Autodesk Fusion 360 part; units mm, degrees
(part 18 of 20)
  spline S542 degree 3 poles (32.1624, -86.398) (32.3125, -86.213) (32.6036, -85.8545) (33.0601, -85.7933) (33.281, -85.7636) knots 0 0 0 0 0.068625 0.133023 0.133023 0.133023 0.133023
  spline S543 degree 3 poles (33.281, -85.7636) (33.4461, -85.772) (33.754, -85.7877) (33.9971, -85.9751) (34.1098, -86.0621) knots 0 0 0 0 0.048244 0.08997 0.08997 0.08997 0.08997
  spline S544 degree 3 poles (34.1098, -86.0621) (34.1941, -86.1844) (34.3835, -86.4593) (34.394, -86.7949) (34.3997, -86.9812) knots 0 0 0 0 0.043695 0.098195 0.098195 0.098195 0.098195
  line L449 (34.3997, -86.9812) -> (34.3997, -89.4676)
  line L450 (34.3997, -89.4676) -> (33.7892, -89.4676)
  line L451 (33.7892, -89.4676) -> (33.7892, -87.1859)
  spline S545 degree 3 poles (33.7892, -87.1859) (33.7892, -87.0797) (33.7892, -86.9003) (33.7468, -86.7264) (33.7295, -86.6555) knots 0 0 0 0 0.031711 0.053535 0.053535 0.053535 0.053535
  spline S546 degree 3 poles (33.7295, -86.6555) (33.7051, -86.6038) (33.6553, -86.4984) (33.561, -86.4297) (33.513, -86.3946) knots 0 0 0 0 0.016863 0.034394 0.034394 0.034394 0.034394
  spline S547 degree 3 poles (33.513, -86.3946) (33.4572, -86.3658) (33.3418, -86.306) (33.2118, -86.2992) (33.1446, -86.2957) knots 0 0 0 0 0.018597 0.038532 0.038532 0.038532 0.038532
  spline S548 degree 3 poles (33.1446, -86.2957) (33.0235, -86.3055) (32.7855, -86.3247) (32.6009, -86.4757) (32.5102, -86.5498) knots 0 0 0 0 0.035532 0.069798 0.069798 0.069798 0.069798
  spline S549 degree 3 poles (32.5102, -86.5498) (32.4369, -86.6565) (32.2698, -86.8996) (32.2621, -87.1966) (32.2578, -87.3632) knots 0 0 0 0 0.038079 0.086792 0.086792 0.086792 0.086792
  line L452 (32.2578, -87.3632) -> (32.2579, -89.4676)
  line L453 (32.2579, -89.4676) -> (31.6439, -89.4676)
  line L454 (31.6439, -89.4676) -> (31.6439, -87.1142)
  spline S550 degree 3 poles (31.6439, -87.1142) (31.6415, -86.9922) (31.6372, -86.7754) (31.5375, -86.584) (31.4939, -86.5003) knots 0 0 0 0 0.036008 0.063954 0.063954 0.063954 0.063954
  spline S551 degree 3 poles (31.4939, -86.5003) (31.4316, -86.4408) (31.2954, -86.3104) (31.1058, -86.3009) (31.0027, -86.2957) knots 0 0 0 0 0.025037 0.054812 0.054812 0.054812 0.054812
  spline S552 degree 3 poles (31.0027, -86.2957) (30.918, -86.3014) (30.7485, -86.3127) (30.5985, -86.3923) (30.5235, -86.4321) knots 0 0 0 0 0.025172 0.050327 0.050327 0.050327 0.050327
  spline S553 degree 3 poles (30.5235, -86.4321) (30.4549, -86.4838) (30.3146, -86.5894) (30.2418, -86.7494) (30.2046, -86.8312) knots 0 0 0 0 0.025339 0.051812 0.051812 0.051812 0.051812
  spline S554 degree 3 poles (30.2046, -86.8312) (30.1759, -86.9375) (30.1091, -87.185) (30.107, -87.4418) (30.1057, -87.5883) knots 0 0 0 0 0.032907 0.076633 0.076633 0.076633 0.076633
  line L455 (30.1057, -87.5883) -> (30.1057, -89.4676)
  line L456 (30.1057, -89.4676) -> (29.4918, -89.4676)
  line L457 (18.1003, -85.1224) -> (18.1003, -84.5324)
  line L458 (18.1003, -84.5324) -> (21.337, -84.5324)
  line L459 (21.337, -84.5324) -> (21.337, -85.0099)
  spline S555 degree 3 poles (21.337, -85.0099) (21.1728, -85.2031) (20.8154, -85.6236) (20.5396, -86.1019) (20.3905, -86.3605) knots 0 0 0 0 0.075903 0.165223 0.165223 0.165223 0.165223
  spline S556 degree 3 poles (20.3905, -86.3605) (20.2435, -86.6418) (19.9525, -87.1986) (19.7607, -87.797) (19.6658, -88.0931) knots 0 0 0 0 0.095012 0.188116 0.188116 0.188116 0.188116
  spline S557 degree 3 poles (19.6658, -88.0931) (19.6097, -88.3112) (19.4935, -88.7629) (19.4519, -89.2274) (19.4304, -89.4676) knots 0 0 0 0 0.06745 0.139654 0.139654 0.139654 0.139654
  line L460 (19.4304, -89.4676) -> (18.7995, -89.4676)
  spline S558 degree 3 poles (18.7995, -89.4676) (18.8147, -89.2495) (18.8485, -88.7675) (18.9667, -88.2987) (19.0314, -88.0419) knots 0 0 0 0 0.065448 0.144689 0.144689 0.144689 0.144689
  spline S559 degree 3 poles (19.0314, -88.0419) (19.1136, -87.7653) (19.2788, -87.2097) (19.5375, -86.6909) (19.6675, -86.4304) knots 0 0 0 0 0.086392 0.173544 0.173544 0.173544 0.173544
  spline S560 degree 3 poles (19.6675, -86.4304) (19.8031, -86.1874) (20.0603, -85.7265) (20.3922, -85.3163) (20.5491, -85.1224) knots 0 0 0 0 0.083307 0.157996 0.157996 0.157996 0.157996
  line L461 (20.5491, -85.1224) -> (18.1003, -85.1224)
  line L462 (29.4918, -139.5) -> (29.4918, -135.8779)
  line L463 (29.4918, -135.8779) -> (30.0409, -135.8779)
  line L464 (30.0409, -135.8779) -> (30.0409, -136.3861)
  spline S561 degree 3 poles (30.0409, -136.3861) (30.1028, -136.3015) (30.2277, -136.131) (30.4051, -136.016) (30.4945, -135.9581) knots 0 0 0 0 0.031158 0.062835 0.062835 0.062835 0.062835
  spline S562 degree 3 poles (30.4945, -135.9581) (30.5937, -135.9108) (30.7976, -135.8137) (31.0232, -135.802) (31.1391, -135.7961) knots 0 0 0 0 0.032617 0.067048 0.067048 0.067048 0.067048
  spline S563 degree 3 poles (31.1391, -135.7961) (31.2636, -135.8008) (31.496, -135.8096) (31.703, -135.9145) (31.7991, -135.9632) knots 0 0 0 0 0.036859 0.068796 0.068796 0.068796 0.068796
  spline S564 degree 3 poles (31.7991, -135.9632) (31.8788, -136.0249) (32.0397, -136.1496) (32.1212, -136.3362) (32.1623, -136.4304) knots 0 0 0 0 0.029725 0.060035 0.060035 0.060035 0.060035
  spline S565 degree 3 poles (32.1623, -136.4304) (32.3125, -136.2455) (32.6036, -135.8869) (33.0601, -135.8257) (33.281, -135.7961) knots 0 0 0 0 0.068625 0.133023 0.133023 0.133023 0.133023
  spline S566 degree 3 poles (33.281, -135.7961) (33.4461, -135.8045) (33.754, -135.8201) (33.9971, -136.0076) (34.1098, -136.0945) knots 0 0 0 0 0.048244 0.08997 0.08997 0.08997 0.08997
  spline S567 degree 3 poles (34.1098, -136.0945) (34.1941, -136.2168) (34.3835, -136.4917) (34.3939, -136.8274) (34.3997, -137.0137) knots 0 0 0 0 0.043695 0.098195 0.098195 0.098195 0.098195
  line L465 (34.3997, -137.0137) -> (34.3997, -139.5)
  line L466 (34.3997, -139.5) -> (33.7892, -139.5)
  line L467 (33.7892, -139.5) -> (33.7892, -137.2183)
  spline S568 degree 3 poles (33.7892, -137.2183) (33.7892, -137.1121) (33.7891, -136.9328) (33.7468, -136.7588) (33.7295, -136.6879) knots 0 0 0 0 0.031711 0.053535 0.053535 0.053535 0.053535
  spline S569 degree 3 poles (33.7295, -136.6879) (33.7051, -136.6363) (33.6552, -136.5309) (33.561, -136.4621) (33.5129, -136.427) knots 0 0 0 0 0.016863 0.034394 0.034394 0.034394 0.034394
  spline S570 degree 3 poles (33.5129, -136.427) (33.4572, -136.3982) (33.3418, -136.3384) (33.2118, -136.3316) (33.1446, -136.3281) knots 0 0 0 0 0.018597 0.038532 0.038532 0.038532 0.038532
  spline S571 degree 3 poles (33.1446, -136.3281) (33.0235, -136.3379) (32.7855, -136.3572) (32.6009, -136.5081) (32.5102, -136.5822) knots 0 0 0 0 0.035532 0.069798 0.069798 0.069798 0.069798
  spline S572 degree 3 poles (32.5102, -136.5822) (32.4369, -136.6889) (32.2697, -136.9321) (32.2621, -137.229) (32.2578, -137.3956) knots 0 0 0 0 0.038079 0.086792 0.086792 0.086792 0.086792
  line L468 (32.2578, -137.3956) -> (32.2578, -139.5)
  line L469 (32.2578, -139.5) -> (31.6439, -139.5)
  line L470 (31.6439, -139.5) -> (31.6439, -137.1467)
  spline S573 degree 3 poles (31.6439, -137.1467) (31.6415, -137.0246) (31.6372, -136.8078) (31.5374, -136.6164) (31.4938, -136.5328) knots 0 0 0 0 0.036008 0.063954 0.063954 0.063954 0.063954
  spline S574 degree 3 poles (31.4938, -136.5328) (31.4316, -136.4732) (31.2954, -136.3428) (31.1057, -136.3333) (31.0027, -136.3281) knots 0 0 0 0 0.025037 0.054812 0.054812 0.054812 0.054812
  spline S575 degree 3 poles (31.0027, -136.3281) (30.918, -136.3338) (30.7485, -136.3451) (30.5985, -136.4247) (30.5235, -136.4645) knots 0 0 0 0 0.025172 0.050327 0.050327 0.050327 0.050327
  spline S576 degree 3 poles (30.5235, -136.4645) (30.4549, -136.5162) (30.3146, -136.6218) (30.2418, -136.7818) (30.2046, -136.8636) knots 0 0 0 0 0.025339 0.051812 0.051812 0.051812 0.051812
  spline S577 degree 3 poles (30.2046, -136.8636) (30.1759, -136.9699) (30.1091, -137.2174) (30.1069, -137.4742) (30.1057, -137.6207) knots 0 0 0 0 0.032907 0.076633 0.076633 0.076633 0.076633
  line L471 (30.1057, -137.6207) -> (30.1057, -139.5)
  line L472 (30.1057, -139.5) -> (29.4918, -139.5)
  line L473 (18.1003, -135.1548) -> (18.1003, -134.5648)
  line L474 (18.1003, -134.5648) -> (21.337, -134.5648)
  line L475 (21.337, -134.5648) -> (21.337, -135.0423)
  spline S578 degree 3 poles (21.337, -135.0423) (21.1728, -135.2355) (20.8153, -135.656) (20.5396, -136.1343) (20.3905, -136.3929) knots 0 0 0 0 0.075903 0.165223 0.165223 0.165223 0.165223
  spline S579 degree 3 poles (20.3905, -136.3929) (20.2435, -136.6742) (19.9525, -137.2311) (19.7607, -137.8294) (19.6657, -138.1255) knots 0 0 0 0 0.095012 0.188116 0.188116 0.188116 0.188116
  spline S580 degree 3 poles (19.6657, -138.1255) (19.6096, -138.3436) (19.4935, -138.7953) (19.4519, -139.2598) (19.4304, -139.5) knots 0 0 0 0 0.06745 0.139654 0.139654 0.139654 0.139654
  line L476 (19.4304, -139.5) -> (18.7994, -139.5)
  spline S581 degree 3 poles (18.7994, -139.5) (18.8147, -139.282) (18.8485, -138.7999) (18.9666, -138.3311) (19.0314, -138.0744) knots 0 0 0 0 0.065448 0.144689 0.144689 0.144689 0.144689
  spline S582 degree 3 poles (19.0314, -138.0744) (19.1136, -137.7977) (19.2788, -137.2421) (19.5375, -136.7233) (19.6674, -136.4628) knots 0 0 0 0 0.086392 0.173544 0.173544 0.173544 0.173544
  spline S583 degree 3 poles (19.6674, -136.4628) (19.8031, -136.2198) (20.0602, -135.7589) (20.3922, -135.3487) (20.5491, -135.1548) knots 0 0 0 0 0.083307 0.157996 0.157996 0.157996 0.157996
  line L477 (20.5491, -135.1548) -> (18.1003, -135.1548)
  line L478 (29.5259, -189.5) -> (29.5259, -185.8779)
  line L479 (29.5259, -185.8779) -> (30.075, -185.8779)
  line L480 (30.075, -185.8779) -> (30.075, -186.3861)
  spline S584 degree 3 poles (30.075, -186.3861) (30.137, -186.3015) (30.2618, -186.131) (30.4392, -186.016) (30.5287, -185.958) knots 0 0 0 0 0.031158 0.062835 0.062835 0.062835 0.062835
  spline S585 degree 3 poles (30.5287, -185.958) (30.6278, -185.9108) (30.8317, -185.8137) (31.0574, -185.802) (31.1733, -185.796) knots 0 0 0 0 0.032617 0.067048 0.067048 0.067048 0.067048
  spline S586 degree 3 poles (31.1733, -185.796) (31.2978, -185.8008) (31.5301, -185.8096) (31.7371, -185.9145) (31.8332, -185.9632) knots 0 0 0 0 0.036859 0.068796 0.068796 0.068796 0.068796
  spline S587 degree 3 poles (31.8332, -185.9632) (31.9129, -186.0249) (32.0738, -186.1496) (32.1553, -186.3362) (32.1965, -186.4304) knots 0 0 0 0 0.029725 0.060035 0.060035 0.060035 0.060035
  spline S588 degree 3 poles (32.1965, -186.4304) (32.3466, -186.2454) (32.6378, -185.8869) (33.0942, -185.8257) (33.3151, -185.796) knots 0 0 0 0 0.068625 0.133023 0.133023 0.133023 0.133023
  spline S589 degree 3 poles (33.3151, -185.796) (33.4802, -185.8045) (33.7881, -185.8201) (34.0312, -186.0076) (34.1439, -186.0945) knots 0 0 0 0 0.048244 0.08997 0.08997 0.08997 0.08997
  spline S590 degree 3 poles (34.1439, -186.0945) (34.2282, -186.2168) (34.4177, -186.4917) (34.4281, -186.8273) (34.4338, -187.0136) knots 0 0 0 0 0.043695 0.098195 0.098195 0.098195 0.098195
  line L481 (34.4338, -187.0136) -> (34.4338, -189.5)
  line L482 (34.4338, -189.5) -> (33.8233, -189.5)
  line L483 (33.8233, -189.5) -> (33.8233, -187.2183)
  spline S591 degree 3 poles (33.8233, -187.2183) (33.8233, -187.1121) (33.8233, -186.9327) (33.7809, -186.7588) (33.7636, -186.6879) knots 0 0 0 0 0.031711 0.053535 0.053535 0.053535 0.053535
  spline S592 degree 3 poles (33.7636, -186.6879) (33.7392, -186.6362) (33.6894, -186.5308) (33.5951, -186.4621) (33.5471, -186.427) knots 0 0 0 0 0.016863 0.034394 0.034394 0.034394 0.034394
  spline S593 degree 3 poles (33.5471, -186.427) (33.4914, -186.3982) (33.3759, -186.3384) (33.246, -186.3316) (33.1787, -186.3281) knots 0 0 0 0 0.018597 0.038532 0.038532 0.038532 0.038532
  spline S594 degree 3 poles (33.1787, -186.3281) (33.0576, -186.3379) (32.8196, -186.3571) (32.635, -186.5081) (32.5443, -186.5822) knots 0 0 0 0 0.035532 0.069798 0.069798 0.069798 0.069798
  spline S595 degree 3 poles (32.5443, -186.5822) (32.471, -186.6889) (32.3039, -186.932) (32.2962, -187.229) (32.292, -187.3956) knots 0 0 0 0 0.038079 0.086792 0.086792 0.086792 0.086792
  line L484 (32.292, -187.3956) -> (32.292, -189.5)
  line L485 (32.292, -189.5) -> (31.678, -189.5)
  line L486 (31.678, -189.5) -> (31.678, -187.1467)
  spline S596 degree 3 poles (31.678, -187.1467) (31.6756, -187.0246) (31.6713, -186.8078) (31.5716, -186.6164) (31.528, -186.5327) knots 0 0 0 0 0.036008 0.063954 0.063954 0.063954 0.063954
  spline S597 degree 3 poles (31.528, -186.5327) (31.4658, -186.4732) (31.3295, -186.3428) (31.1399, -186.3333) (31.0368, -186.3281) knots 0 0 0 0 0.025037 0.054812 0.054812 0.054812 0.054812
  spline S598 degree 3 poles (31.0368, -186.3281) (30.9521, -186.3338) (30.7826, -186.3451) (30.6326, -186.4247) (30.5576, -186.4645) knots 0 0 0 0 0.025172 0.050327 0.050327 0.050327 0.050327
  spline S599 degree 3 poles (30.5576, -186.4645) (30.489, -186.5162) (30.3487, -186.6218) (30.2759, -186.7818) (30.2388, -186.8636) knots 0 0 0 0 0.025339 0.051812 0.051812 0.051812 0.051812
  spline S600 degree 3 poles (30.2388, -186.8636) (30.21, -186.9699) (30.1432, -187.2174) (30.1411, -187.4742) (30.1398, -187.6207) knots 0 0 0 0 0.032907 0.076633 0.076633 0.076633 0.076633
  line L487 (30.1398, -187.6207) -> (30.1398, -189.5)
  line L488 (30.1398, -189.5) -> (29.5259, -189.5)
  line L489 (21.279, -185.7244) -> (20.6685, -185.7722)
  spline S601 degree 3 poles (20.6685, -185.7722) (20.6425, -185.6649) (20.5967, -185.4753) (20.485, -185.3161) (20.4366, -185.2469) knots 0 0 0 0 0.032737 0.057863 0.057863 0.057863 0.057863
  spline S602 degree 3 poles (20.4366, -185.2469) (20.3486, -185.1703) (20.1722, -185.0168) (19.9394, -184.9952) (19.8227, -184.9843) knots 0 0 0 0 0.034068 0.068298 0.068298 0.068298 0.068298
  spline S603 degree 3 poles (19.8227, -184.9843) (19.7285, -184.9907) (19.5433, -185.0032) (19.3853, -185.1003) (19.3076, -185.148) knots 0 0 0 0 0.027843 0.054766 0.054766 0.054766 0.054766
  spline S604 degree 3 poles (19.3076, -185.148) (19.2148, -185.2299) (19.0188, -185.4028) (18.9086, -185.6403) (18.8506, -185.7654) knots 0 0 0 0 0.036718 0.077555 0.077555 0.077555 0.077555
  spline S605 degree 3 poles (18.8506, -185.7654) (18.8017, -185.9283) (18.6886, -186.3047) (18.681, -186.6983) (18.6767, -186.9216) knots 0 0 0 0 0.050812 0.1174 0.1174 0.1174 0.1174
  spline S606 degree 3 poles (18.6767, -186.9216) (18.753, -186.8171) (18.9011, -186.6144) (19.1152, -186.4836) (19.219, -186.4202) knots 0 0 0 0 0.038374 0.074495 0.074495 0.074495 0.074495
  spline S607 degree 3 poles (19.219, -186.4202) (19.3267, -186.3724) (19.5409, -186.2776) (19.7747, -186.2635) (19.8909, -186.2565) knots 0 0 0 0 0.035048 0.069654 0.069654 0.069654 0.069654
  spline S608 degree 3 poles (19.8909, -186.2565) (20.0883, -186.2757) (20.485, -186.3143) (20.7853, -186.5766) (20.9362, -186.7084) knots 0 0 0 0 0.057942 0.116462 0.116462 0.116462 0.116462
  spline S609 degree 3 poles (20.9362, -186.7084) (21.062, -186.8743) (21.3235, -187.2192) (21.3526, -187.6519) (21.3677, -187.8765) knots 0 0 0 0 0.061076 0.12698 0.12698 0.12698 0.12698
  spline S610 degree 3 poles (21.3677, -187.8765) (21.3596, -188.0299) (21.3435, -188.3336) (21.2239, -188.6131) (21.1647, -188.7514) knots 0 0 0 0 0.045687 0.090433 0.090433 0.090433 0.090433
  spline S611 degree 3 poles (21.1647, -188.7514) (21.0922, -188.8773) (20.9503, -189.1236) (20.7197, -189.2894) (20.6071, -189.3704) knots 0 0 0 0 0.043053 0.084173 0.084173 0.084173 0.084173
  spline S612 degree 3 poles (20.6071, -189.3704) (20.4833, -189.4331) (20.2303, -189.5612) (19.9469, -189.5771) (19.8022, -189.5853) knots 0 0 0 0 0.041145 0.084115 0.084115 0.084115 0.084115
  spline S613 degree 3 poles (19.8022, -189.5853) (19.5589, -189.5626) (19.0767, -189.5177) (18.7248, -189.1854) (18.5505, -189.0208) knots 0 0 0 0 0.071077 0.140887 0.140887 0.140887 0.140887
  spline S614 degree 3 poles (18.5505, -189.0208) (18.41, -188.7773) (18.0802, -188.2056) (18.0713, -187.5415) (18.0662, -187.1603) knots 0 0 0 0 0.083095 0.195067 0.195067 0.195067 0.195067
  spline S615 degree 3 poles (18.0662, -187.1603) (18.0727, -186.7324) (18.084, -185.9831) (18.4463, -185.3319) (18.6016, -185.0525) knots 0 0 0 0 0.125884 0.220443 0.220443 0.220443 0.220443
  spline S616 degree 3 poles (18.6016, -185.0525) (18.7734, -184.8854) (19.1238, -184.5445) (19.6115, -184.5015) (19.8602, -184.4795) knots 0 0 0 0 0.069661 0.142118 0.142118 0.142118 0.142118
  spline S617 degree 3 poles (19.8602, -184.4795) (20.0449, -184.4907) (20.3984, -184.512) (20.6885, -184.7139) (20.8271, -184.8104) knots 0 0 0 0 0.054308 0.103968 0.103968 0.103968 0.103968
  spline S618 degree 3 poles (20.8271, -184.8104) (20.9406, -184.9351) (21.178, -185.196) (21.2444, -185.5432) (21.279, -185.7244) knots 0 0 0 0 0.049602 0.103747 0.103747 0.103747 0.103747
  line L490 (29.5256, -239.5001) -> (29.5256, -235.878)
  line L491 (29.5256, -235.878) -> (30.0747, -235.878)
  line L492 (30.0747, -235.878) -> (30.0747, -236.3862)
  spline S619 degree 3 poles (30.0747, -236.3862) (30.1366, -236.3016) (30.2615, -236.1311) (30.4389, -236.0161) (30.5283, -235.9582) knots 0 0 0 0 0.031158 0.062835 0.062835 0.062835 0.062835
  spline S620 degree 3 poles (30.5283, -235.9582) (30.6275, -235.9109) (30.8314, -235.8138) (31.0571, -235.8022) (31.173, -235.7962) knots 0 0 0 0 0.032617 0.067048 0.067048 0.067048 0.067048
  spline S621 degree 3 poles (31.173, -235.7962) (31.2975, -235.8009) (31.5298, -235.8098) (31.7368, -235.9146) (31.8329, -235.9633) knots 0 0 0 0 0.036859 0.068796 0.068796 0.068796 0.068796
  spline S622 degree 3 poles (31.8329, -235.9633) (31.9126, -236.025) (32.0735, -236.1497) (32.155, -236.3363) (32.1961, -236.4305) knots 0 0 0 0 0.029725 0.060035 0.060035 0.060035 0.060035
  spline S623 degree 3 poles (32.1961, -236.4305) (32.3463, -236.2456) (32.6374, -235.887) (33.0939, -235.8258) (33.3148, -235.7962) knots 0 0 0 0 0.068625 0.133023 0.133023 0.133023 0.133023
  spline S624 degree 3 poles (33.3148, -235.7962) (33.4799, -235.8046) (33.7878, -235.8203) (34.0309, -236.0077) (34.1436, -236.0946) knots 0 0 0 0 0.048244 0.08997 0.08997 0.08997 0.08997
  spline S625 degree 3 poles (34.1436, -236.0946) (34.2279, -236.2169) (34.4173, -236.4919) (34.4277, -236.8275) (34.4335, -237.0138) knots 0 0 0 0 0.043695 0.098195 0.098195 0.098195 0.098195
  line L493 (34.4335, -237.0138) -> (34.4335, -239.5001)
  line L494 (34.4335, -239.5001) -> (33.823, -239.5001)
  line L495 (33.823, -239.5001) -> (33.823, -237.2184)
  spline S626 degree 3 poles (33.823, -237.2184) (33.823, -237.1122) (33.8229, -236.9329) (33.7806, -236.759) (33.7633, -236.6881) knots 0 0 0 0 0.031711 0.053535 0.053535 0.053535 0.053535
  spline S627 degree 3 poles (33.7633, -236.6881) (33.7389, -236.6364) (33.6891, -236.531) (33.5948, -236.4622) (33.5468, -236.4271) knots 0 0 0 0 0.016863 0.034394 0.034394 0.034394 0.034394
  spline S628 degree 3 poles (33.5468, -236.4271) (33.491, -236.3983) (33.3756, -236.3386) (33.2456, -236.3318) (33.1784, -236.3282) knots 0 0 0 0 0.018597 0.038532 0.038532 0.038532 0.038532
  spline S629 degree 3 poles (33.1784, -236.3282) (33.0573, -236.338) (32.8193, -236.3573) (32.6347, -236.5082) (32.544, -236.5823) knots 0 0 0 0 0.035532 0.069798 0.069798 0.069798 0.069798
  spline S630 degree 3 poles (32.544, -236.5823) (32.4707, -236.689) (32.3035, -236.9322) (32.2959, -237.2291) (32.2916, -237.3958) knots 0 0 0 0 0.038079 0.086792 0.086792 0.086792 0.086792
  line L496 (32.2916, -237.3958) -> (32.2916, -239.5001)
  line L497 (32.2916, -239.5001) -> (31.6777, -239.5001)
  line L498 (31.6777, -239.5001) -> (31.6777, -237.1468)
  spline S631 degree 3 poles (31.6777, -237.1468) (31.6753, -237.0247) (31.671, -236.808) (31.5713, -236.6165) (31.5277, -236.5329) knots 0 0 0 0 0.036008 0.063954 0.063954 0.063954 0.063954
  spline S632 degree 3 poles (31.5277, -236.5329) (31.4654, -236.4733) (31.3292, -236.3429) (31.1396, -236.3334) (31.0365, -236.3282) knots 0 0 0 0 0.025037 0.054812 0.054812 0.054812 0.054812
  spline S633 degree 3 poles (31.0365, -236.3282) (30.9518, -236.3339) (30.7823, -236.3452) (30.6323, -236.4249) (30.5573, -236.4646) knots 0 0 0 0 0.025172 0.050327 0.050327 0.050327 0.050327
  spline S634 degree 3 poles (30.5573, -236.4646) (30.4887, -236.5163) (30.3484, -236.6219) (30.2756, -236.7819) (30.2384, -236.8637) knots 0 0 0 0 0.025339 0.051812 0.051812 0.051812 0.051812
  spline S635 degree 3 poles (30.2384, -236.8637) (30.2097, -236.97) (30.1429, -237.2175) (30.1407, -237.4743) (30.1395, -237.6208) knots 0 0 0 0 0.032907 0.076633 0.076633 0.076633 0.076633
  line L499 (30.1395, -237.6208) -> (30.1395, -239.5001)
  line L500 (30.1395, -239.5001) -> (29.5256, -239.5001)
  line L501 (21.2787, -235.7245) -> (20.6682, -235.7722)
  spline S636 degree 3 poles (20.6682, -235.7722) (20.6422, -235.6649) (20.5964, -235.4754) (20.4847, -235.3161) (20.4363, -235.247) knots 0 0 0 0 0.032737 0.057863 0.057863 0.057863 0.057863
  spline S637 degree 3 poles (20.4363, -235.247) (20.3483, -235.1704) (20.1719, -235.0168) (19.9391, -234.9952) (19.8223, -234.9843) knots 0 0 0 0 0.034068 0.068298 0.068298 0.068298 0.068298
  spline S638 degree 3 poles (19.8223, -234.9843) (19.7282, -234.9907) (19.543, -235.0032) (19.385, -235.1003) (19.3073, -235.148) knots 0 0 0 0 0.027843 0.054766 0.054766 0.054766 0.054766
  spline S639 degree 3 poles (19.3073, -235.148) (19.2145, -235.2299) (19.0185, -235.4028) (18.9083, -235.6403) (18.8503, -235.7654) knots 0 0 0 0 0.036718 0.077555 0.077555 0.077555 0.077555
  spline S640 degree 3 poles (18.8503, -235.7654) (18.8014, -235.9283) (18.6883, -236.3047) (18.6807, -236.6983) (18.6764, -236.9216) knots 0 0 0 0 0.050812 0.1174 0.1174 0.1174 0.1174
  spline S641 degree 3 poles (18.6764, -236.9216) (18.7527, -236.8172) (18.9008, -236.6145) (19.1149, -236.4836) (19.2187, -236.4202) knots 0 0 0 0 0.038374 0.074495 0.074495 0.074495 0.074495
  spline S642 degree 3 poles (19.2187, -236.4202) (19.3264, -236.3725) (19.5406, -236.2776) (19.7744, -236.2635) (19.8906, -236.2565) knots 0 0 0 0 0.035048 0.069654 0.069654 0.069654 0.069654
  spline S643 degree 3 poles (19.8906, -236.2565) (20.0879, -236.2757) (20.4847, -236.3143) (20.785, -236.5766) (20.9359, -236.7084) knots 0 0 0 0 0.057942 0.116462 0.116462 0.116462 0.116462
  spline S644 degree 3 poles (20.9359, -236.7084) (21.0617, -236.8743) (21.3232, -237.2192) (21.3523, -237.652) (21.3673, -237.8766) knots 0 0 0 0 0.061076 0.12698 0.12698 0.12698 0.12698
  spline S645 degree 3 poles (21.3673, -237.8766) (21.3592, -238.03) (21.3432, -238.3336) (21.2236, -238.6131) (21.1644, -238.7514) knots 0 0 0 0 0.045687 0.090433 0.090433 0.090433 0.090433
  spline S646 degree 3 poles (21.1644, -238.7514) (21.0919, -238.8774) (20.95, -239.1236) (20.7194, -239.2894) (20.6068, -239.3704) knots 0 0 0 0 0.043053 0.084173 0.084173 0.084173 0.084173
  spline S647 degree 3 poles (20.6068, -239.3704) (20.483, -239.4331) (20.2299, -239.5612) (19.9466, -239.5771) (19.8018, -239.5853) knots 0 0 0 0 0.041145 0.084115 0.084115 0.084115 0.084115
  spline S648 degree 3 poles (19.8018, -239.5853) (19.5586, -239.5626) (19.0764, -239.5177) (18.7245, -239.1855) (18.5501, -239.0208) knots 0 0 0 0 0.071077 0.140887 0.140887 0.140887 0.140887
  spline S649 degree 3 poles (18.5501, -239.0208) (18.4097, -238.7773) (18.0799, -238.2056) (18.071, -237.5415) (18.0659, -237.1603) knots 0 0 0 0 0.083095 0.195067 0.195067 0.195067 0.195067
  spline S650 degree 3 poles (18.0659, -237.1603) (18.0723, -236.7324) (18.0837, -235.9831) (18.4459, -235.3319) (18.6013, -235.0525) knots 0 0 0 0 0.125884 0.220443 0.220443 0.220443 0.220443
  spline S651 degree 3 poles (18.6013, -235.0525) (18.7731, -234.8854) (19.1235, -234.5445) (19.6112, -234.5015) (19.8599, -234.4796) knots 0 0 0 0 0.069661 0.142118 0.142118 0.142118 0.142118
  spline S652 degree 3 poles (19.8599, -234.4796) (20.0446, -234.4907) (20.3981, -234.5121) (20.6882, -234.714) (20.8268, -234.8104) knots 0 0 0 0 0.054308 0.103968 0.103968 0.103968 0.103968
  spline S653 degree 3 poles (20.8268, -234.8104) (20.9403, -234.9351) (21.1777, -235.196) (21.2441, -235.5432) (21.2787, -235.7245) knots 0 0 0 0 0.049602 0.103747 0.103747 0.103747 0.103747
  line L502 (29.5124, -289.4659) -> (29.5124, -285.8438)
  line L503 (29.5124, -285.8438) -> (30.0615, -285.8438)
  line L504 (30.0615, -285.8438) -> (30.0615, -286.3519)
  spline S654 degree 3 poles (30.0615, -286.3519) (30.1234, -286.2674) (30.2483, -286.0968) (30.4257, -285.9819) (30.5151, -285.9239) knots 0 0 0 0 0.031158 0.062835 0.062835 0.062835 0.062835
  spline S655 degree 3 poles (30.5151, -285.9239) (30.6143, -285.8767) (30.8182, -285.7796) (31.0438, -285.7679) (31.1597, -285.7619) knots 0 0 0 0 0.032617 0.067048 0.067048 0.067048 0.067048
  spline S656 degree 3 poles (31.1597, -285.7619) (31.2842, -285.7666) (31.5166, -285.7755) (31.7236, -285.8803) (31.8197, -285.929) knots 0 0 0 0 0.036859 0.068796 0.068796 0.068796 0.068796
  spline S657 degree 3 poles (31.8197, -285.929) (31.8994, -285.9907) (32.0603, -286.1154) (32.1418, -286.302) (32.1829, -286.3963) knots 0 0 0 0 0.029725 0.060035 0.060035 0.060035 0.060035
  spline S658 degree 3 poles (32.1829, -286.3963) (32.3331, -286.2113) (32.6242, -285.8528) (33.0806, -285.7915) (33.3016, -285.7619) knots 0 0 0 0 0.068625 0.133023 0.133023 0.133023 0.133023
  spline S659 degree 3 poles (33.3016, -285.7619) (33.4667, -285.7703) (33.7746, -285.786) (34.0177, -285.9734) (34.1304, -286.0603) knots 0 0 0 0 0.048244 0.08997 0.08997 0.08997 0.08997
  spline S660 degree 3 poles (34.1304, -286.0603) (34.2147, -286.1826) (34.4041, -286.4576) (34.4145, -286.7932) (34.4203, -286.9795) knots 0 0 0 0 0.043695 0.098195 0.098195 0.098195 0.098195
  line L505 (34.4203, -286.9795) -> (34.4203, -289.4658)
  line L506 (34.4203, -289.4658) -> (33.8098, -289.4658)
  line L507 (33.8098, -289.4658) -> (33.8098, -287.1841)
  spline S661 degree 3 poles (33.8098, -287.1841) (33.8098, -287.0779) (33.8097, -286.8986) (33.7674, -286.7247) (33.7501, -286.6538) knots 0 0 0 0 0.031711 0.053535 0.053535 0.053535 0.053535
  spline S662 degree 3 poles (33.7501, -286.6538) (33.7257, -286.6021) (33.6758, -286.4967) (33.5816, -286.4279) (33.5335, -286.3929) knots 0 0 0 0 0.016863 0.034394 0.034394 0.034394 0.034394
  spline S663 degree 3 poles (33.5335, -286.3929) (33.4778, -286.364) (33.3624, -286.3043) (33.2324, -286.2975) (33.1652, -286.294) knots 0 0 0 0 0.018597 0.038532 0.038532 0.038532 0.038532
  spline S664 degree 3 poles (33.1652, -286.294) (33.044, -286.3038) (32.8061, -286.323) (32.6215, -286.4739) (32.5308, -286.548) knots 0 0 0 0 0.035532 0.069798 0.069798 0.069798 0.069798
  spline S665 degree 3 poles (32.5308, -286.548) (32.4575, -286.6547) (32.2903, -286.8979) (32.2827, -287.1948) (32.2784, -287.3615) knots 0 0 0 0 0.038079 0.086792 0.086792 0.086792 0.086792
  line L508 (32.2784, -287.3615) -> (32.2784, -289.4659)
  line L509 (32.2784, -289.4659) -> (31.6645, -289.4659)
  line L510 (31.6645, -289.4659) -> (31.6645, -287.1125)
  spline S666 degree 3 poles (31.6645, -287.1125) (31.6621, -286.9905) (31.6578, -286.7737) (31.558, -286.5822) (31.5144, -286.4986) knots 0 0 0 0 0.036008 0.063954 0.063954 0.063954 0.063954
  spline S667 degree 3 poles (31.5144, -286.4986) (31.4522, -286.439) (31.316, -286.3086) (31.1263, -286.2991) (31.0233, -286.294) knots 0 0 0 0 0.025037 0.054812 0.054812 0.054812 0.054812
  spline S668 degree 3 poles (31.0233, -286.294) (30.9385, -286.2996) (30.7691, -286.311) (30.6191, -286.3906) (30.5441, -286.4304) knots 0 0 0 0 0.025172 0.050327 0.050327 0.050327 0.050327
  spline S669 degree 3 poles (30.5441, -286.4304) (30.4755, -286.482) (30.3352, -286.5877) (30.2624, -286.7477) (30.2252, -286.8294) knots 0 0 0 0 0.025339 0.051812 0.051812 0.051812 0.051812
  spline S670 degree 3 poles (30.2252, -286.8294) (30.1965, -286.9357) (30.1297, -287.1833) (30.1275, -287.4401) (30.1263, -287.5866) knots 0 0 0 0 0.032907 0.076633 0.076633 0.076633 0.076633
  line L511 (30.1263, -287.5866) -> (30.1263, -289.4659)
  line L512 (30.1263, -289.4659) -> (29.5124, -289.4659)
  line L513 (18.0799, -288.1562) -> (18.7245, -288.1016)
  spline S671 degree 3 poles (18.7245, -288.1016) (18.7522, -288.2449) (18.8035, -288.5098) (18.9773, -288.7151) (19.0571, -288.8093) knots 0 0 0 0 0.042908 0.079365 0.079365 0.079365 0.079365
  spline S672 degree 3 poles (19.0571, -288.8093) (19.1493, -288.8785) (19.3359, -289.0184) (19.5686, -289.037) (19.6863, -289.0464) knots 0 0 0 0 0.033826 0.068485 0.068485 0.068485 0.068485
  spline S673 degree 3 poles (19.6863, -289.0464) (19.8288, -289.0321) (20.1156, -289.0033) (20.3292, -288.8096) (20.4367, -288.7121) knots 0 0 0 0 0.041772 0.0841 0.0841 0.0841 0.0841
  spline S674 degree 3 poles (20.4367, -288.7121) (20.5261, -288.5871) (20.7153, -288.3226) (20.7339, -287.997) (20.7436, -287.8254) knots 0 0 0 0 0.045186 0.095569 0.095569 0.095569 0.095569
  spline S675 degree 3 poles (20.7436, -287.8254) (20.7346, -287.663) (20.7175, -287.3567) (20.5346, -287.1117) (20.4486, -286.9966) knots 0 0 0 0 0.047557 0.089725 0.089725 0.089725 0.089725
  spline S676 degree 3 poles (20.4486, -286.9966) (20.3401, -286.9081) (20.1155, -286.7248) (19.8259, -286.7039) (19.6761, -286.693) knots 0 0 0 0 0.040971 0.08482 0.08482 0.08482 0.08482
  spline S677 degree 3 poles (19.6761, -286.693) (19.5805, -286.6982) (19.3931, -286.7082) (19.2236, -286.7885) (19.1406, -286.8278) knots 0 0 0 0 0.028423 0.055689 0.055689 0.055689 0.055689
  spline S678 degree 3 poles (19.1406, -286.8278) (19.0658, -286.8753) (18.9189, -286.9685) (18.8159, -287.1086) (18.7655, -287.1773) knots 0 0 0 0 0.026342 0.051681 0.051681 0.051681 0.051681
  line L514 (18.7655, -287.1773) -> (18.1891, -287.1023)
  line L515 (18.1891, -287.1023) -> (18.6734, -284.5341)
  line L516 (18.6734, -284.5341) -> (21.1597, -284.5341)
  line L517 (21.1597, -284.5341) -> (21.1597, -285.1207)
  line L518 (21.1597, -285.1207) -> (19.1645, -285.1207)
  line L519 (19.1645, -285.1207) -> (18.8951, -286.4645)
  spline S679 degree 3 poles (18.8951, -286.4645) (19.0446, -286.373) (19.3354, -286.195) (19.6748, -286.1652) (19.8398, -286.1507) knots 0 0 0 0 0.051785 0.100763 0.100763 0.100763 0.100763
  spline S680 degree 3 poles (19.8398, -286.1507) (20.049, -286.1691) (20.4647, -286.2056) (20.7855, -286.472) (20.9449, -286.6044) knots 0 0 0 0 0.061424 0.122014 0.122014 0.122014 0.122014
  spline S681 degree 3 poles (20.9449, -286.6044) (21.0761, -286.7698) (21.347, -287.1111) (21.3787, -287.5465) (21.3951, -287.7708) knots 0 0 0 0 0.061868 0.12764 0.12764 0.12764 0.12764
  spline S682 degree 3 poles (21.3951, -287.7708) (21.3799, -287.9877) (21.35, -288.4136) (21.1148, -288.7695) (20.9994, -288.9441) knots 0 0 0 0 0.064036 0.125703 0.125703 0.125703 0.125703
  spline S683 degree 3 poles (20.9994, -288.9441) (20.8217, -289.1211) (20.4586, -289.4828) (19.9473, -289.528) (19.6863, -289.5511) knots 0 0 0 0 0.072854 0.148822 0.148822 0.148822 0.148822
  spline S684 degree 3 poles (19.6863, -289.5511) (19.4731, -289.5384) (19.0656, -289.514) (18.7319, -289.2805) (18.5728, -289.1692) knots 0 0 0 0 0.062678 0.119794 0.119794 0.119794 0.119794
  spline S685 degree 3 poles (18.5728, -289.1692) (18.4441, -289.0288) (18.1799, -288.7404) (18.1138, -288.3544) (18.0799, -288.1562) knots 0 0 0 0 0.055877 0.114795 0.114795 0.114795 0.114795
  line L520 (29.5137, -339.4997) -> (29.5136, -335.8776)
  line L521 (29.5136, -335.8776) -> (30.0628, -335.8776)
  line L522 (30.0628, -335.8776) -> (30.0628, -336.3858)
  spline S686 degree 3 poles (30.0628, -336.3858) (30.1247, -336.3012) (30.2495, -336.1307) (30.4269, -336.0157) (30.5164, -335.9577) knots 0 0 0 0 0.031158 0.062835 0.062835 0.062835 0.062835
  spline S687 degree 3 poles (30.5164, -335.9577) (30.6156, -335.9105) (30.8194, -335.8134) (31.0451, -335.8017) (31.161, -335.7957) knots 0 0 0 0 0.032617 0.067048 0.067048 0.067048 0.067048
  spline S688 degree 3 poles (31.161, -335.7957) (31.2855, -335.8004) (31.5179, -335.8093) (31.7249, -335.9141) (31.8209, -335.9628) knots 0 0 0 0 0.036859 0.068796 0.068796 0.068796 0.068796
  spline S689 degree 3 poles (31.8209, -335.9628) (31.9006, -336.0245) (32.0615, -336.1492) (32.143, -336.3358) (32.1842, -336.4301) knots 0 0 0 0 0.029725 0.060035 0.060035 0.060035 0.060035
  spline S690 degree 3 poles (32.1842, -336.4301) (32.3344, -336.2451) (32.6255, -335.8865) (33.0819, -335.8253) (33.3029, -335.7956) knots 0 0 0 0 0.068625 0.133023 0.133023 0.133023 0.133023
  spline S691 degree 3 poles (33.3029, -335.7956) (33.468, -335.8041) (33.7758, -335.8197) (34.0189, -336.0071) (34.1317, -336.0941) knots 0 0 0 0 0.048244 0.08997 0.08997 0.08997 0.08997
  spline S692 degree 3 poles (34.1317, -336.0941) (34.216, -336.2164) (34.4054, -336.4913) (34.4158, -336.8269) (34.4216, -337.0132) knots 0 0 0 0 0.043695 0.098195 0.098195 0.098195 0.098195
  line L523 (34.4216, -337.0132) -> (34.4216, -339.4996)
  line L524 (34.4216, -339.4996) -> (33.8111, -339.4996)
  line L525 (33.8111, -339.4996) -> (33.8111, -337.2179)
  spline S693 degree 3 poles (33.8111, -337.2179) (33.8111, -337.1117) (33.811, -336.9323) (33.7687, -336.7584) (33.7514, -336.6875) knots 0 0 0 0 0.031711 0.053535 0.053535 0.053535 0.053535
  spline S694 degree 3 poles (33.7514, -336.6875) (33.7269, -336.6358) (33.6771, -336.5304) (33.5828, -336.4617) (33.5348, -336.4266) knots 0 0 0 0 0.016863 0.034394 0.034394 0.034394 0.034394
  spline S695 degree 3 poles (33.5348, -336.4266) (33.4791, -336.3978) (33.3636, -336.338) (33.2337, -336.3312) (33.1665, -336.3277) knots 0 0 0 0 0.018597 0.038532 0.038532 0.038532 0.038532
  spline S696 degree 3 poles (33.1665, -336.3277) (33.0453, -336.3375) (32.8074, -336.3568) (32.6227, -336.5077) (32.5321, -336.5818) knots 0 0 0 0 0.035532 0.069798 0.069798 0.069798 0.069798
  spline S697 degree 3 poles (32.5321, -336.5818) (32.4588, -336.6885) (32.2916, -336.9317) (32.284, -337.2286) (32.2797, -337.3953) knots 0 0 0 0 0.038079 0.086792 0.086792 0.086792 0.086792
  line L526 (32.2797, -337.3953) -> (32.2798, -339.4996)
  line L527 (32.2798, -339.4996) -> (31.6659, -339.4996)
  line L528 (31.6659, -339.4996) -> (31.6658, -337.1463)
  spline S698 degree 3 poles (31.6658, -337.1463) (31.6634, -337.0243) (31.6591, -336.8075) (31.5593, -336.616) (31.5157, -336.5324) knots 0 0 0 0 0.036008 0.063954 0.063954 0.063954 0.063954
  spline S699 degree 3 poles (31.5157, -336.5324) (31.4535, -336.4728) (31.3173, -336.3424) (31.1276, -336.3329) (31.0246, -336.3278) knots 0 0 0 0 0.025037 0.054812 0.054812 0.054812 0.054812
  spline S700 degree 3 poles (31.0246, -336.3278) (30.9398, -336.3334) (30.7704, -336.3448) (30.6204, -336.4244) (30.5454, -336.4642) knots 0 0 0 0 0.025173 0.050327 0.050327 0.050327 0.050327
  spline S701 degree 3 poles (30.5454, -336.4642) (30.4768, -336.5159) (30.3364, -336.6215) (30.2637, -336.7815) (30.2265, -336.8633) knots 0 0 0 0 0.025339 0.051812 0.051812 0.051812 0.051812
  spline S702 degree 3 poles (30.2265, -336.8633) (30.1978, -336.9696) (30.131, -337.2171) (30.1288, -337.4739) (30.1276, -337.6204) knots 0 0 0 0 0.032907 0.076633 0.076633 0.076633 0.076633
  line L529 (30.1276, -337.6204) -> (30.1277, -339.4997)
  line L530 (30.1277, -339.4997) -> (29.5137, -339.4997)
  line L531 (18.0812, -338.1903) -> (18.7258, -338.1357)
  spline S703 degree 3 poles (18.7258, -338.1357) (18.7536, -338.279) (18.8048, -338.5439) (18.9786, -338.7491) (19.0584, -338.8434) knots 0 0 0 0 0.042908 0.079365 0.079365 0.079365 0.079365
  spline S704 degree 3 poles (19.0584, -338.8434) (19.1506, -338.9125) (19.3372, -339.0525) (19.5699, -339.0711) (19.6877, -339.0804) knots 0 0 0 0 0.033826 0.068485 0.068485 0.068485 0.068485
  spline S705 degree 3 poles (19.6877, -339.0804) (19.8301, -339.0661) (20.1169, -339.0374) (20.3305, -338.8437) (20.438, -338.7462) knots 0 0 0 0 0.041772 0.0841 0.0841 0.0841 0.0841
  spline S706 degree 3 poles (20.438, -338.7462) (20.5275, -338.6211) (20.7167, -338.3566) (20.7352, -338.031) (20.7449, -337.8594) knots 0 0 0 0 0.045186 0.095569 0.095569 0.095569 0.095569
  spline S707 degree 3 poles (20.7449, -337.8594) (20.7359, -337.6971) (20.7188, -337.3908) (20.5359, -337.1458) (20.4499, -337.0306) knots 0 0 0 0 0.047557 0.089725 0.089725 0.089725 0.089725
  spline S708 degree 3 poles (20.4499, -337.0306) (20.3414, -336.9421) (20.1168, -336.7589) (19.8271, -336.7379) (19.6774, -336.7271) knots 0 0 0 0 0.040971 0.08482 0.08482 0.08482 0.08482
  spline S709 degree 3 poles (19.6774, -336.7271) (19.5817, -336.7322) (19.3944, -336.7423) (19.2249, -336.8225) (19.1419, -336.8618) knots 0 0 0 0 0.028423 0.055689 0.055689 0.055689 0.055689
  spline S710 degree 3 poles (19.1419, -336.8618) (19.0671, -336.9094) (18.9202, -337.0026) (18.8172, -337.1427) (18.7667, -337.2114) knots 0 0 0 0 0.026342 0.051681 0.051681 0.051681 0.051681
  line L532 (18.7667, -337.2114) -> (18.1903, -337.1364)
  line L533 (18.1903, -337.1364) -> (18.6746, -334.5682)
  line L534 (18.6746, -334.5682) -> (21.161, -334.5681)
  line L535 (21.161, -334.5681) -> (21.161, -335.1548)
  line L536 (21.161, -335.1548) -> (19.1657, -335.1548)
  line L537 (19.1657, -335.1548) -> (18.8963, -336.4986)
  spline S711 degree 3 poles (18.8963, -336.4986) (19.0458, -336.4071) (19.3367, -336.2291) (19.6761, -336.1993) (19.8411, -336.1848) knots 0 0 0 0 0.051785 0.100763 0.100763 0.100763 0.100763
  spline S712 degree 3 poles (19.8411, -336.1848) (20.0503, -336.2032) (20.4659, -336.2397) (20.7868, -336.5061) (20.9461, -336.6384) knots 0 0 0 0 0.061424 0.122014 0.122014 0.122014 0.122014
  spline S713 degree 3 poles (20.9461, -336.6384) (21.0774, -336.8038) (21.3483, -337.1451) (21.38, -337.5805) (21.3964, -337.8048) knots 0 0 0 0 0.061868 0.12764 0.12764 0.12764 0.12764
  spline S714 degree 3 poles (21.3964, -337.8048) (21.3812, -338.0218) (21.3513, -338.4476) (21.1161, -338.8035) (21.0008, -338.9781) knots 0 0 0 0 0.064036 0.125703 0.125703 0.125703 0.125703
  spline S715 degree 3 poles (21.0008, -338.9781) (20.823, -339.1551) (20.46, -339.5168) (19.9487, -339.5621) (19.6877, -339.5852) knots 0 0 0 0 0.072854 0.148822 0.148822 0.148822 0.148822
  spline S716 degree 3 poles (19.6877, -339.5852) (19.4745, -339.5725) (19.0669, -339.5481) (18.7332, -339.3146) (18.5741, -339.2033) knots 0 0 0 0 0.062678 0.119794 0.119794 0.119794 0.119794
  spline S717 degree 3 poles (18.5741, -339.2033) (18.4455, -339.0629) (18.1812, -338.7745) (18.1151, -338.3885) (18.0812, -338.1903) knots 0 0 0 0 0.055877 0.114795 0.114795 0.114795 0.114795
  line L538 (29.6139, -389.4998) -> (29.6138, -385.8777)
  line L539 (29.6138, -385.8777) -> (30.163, -385.8777)
  line L540 (30.163, -385.8777) -> (30.163, -386.3859)
  spline S718 degree 3 poles (30.163, -386.3859) (30.2249, -386.3013) (30.3497, -386.1308) (30.5271, -386.0158) (30.6166, -385.9579) knots 0 0 0 0 0.031158 0.062835 0.062835 0.062835 0.062835
  spline S719 degree 3 poles (30.6166, -385.9579) (30.7157, -385.9106) (30.9196, -385.8135) (31.1453, -385.8018) (31.2612, -385.7958) knots 0 0 0 0 0.032617 0.067048 0.067048 0.067048 0.067048
  spline S720 degree 3 poles (31.2612, -385.7958) (31.3857, -385.8006) (31.6181, -385.8094) (31.825, -385.9143) (31.9211, -385.963) knots 0 0 0 0 0.036859 0.068796 0.068796 0.068796 0.068796
  spline S721 degree 3 poles (31.9211, -385.963) (32.0008, -386.0247) (32.1617, -386.1493) (32.2432, -386.336) (32.2844, -386.4302) knots 0 0 0 0 0.029725 0.060035 0.060035 0.060035 0.060035
  spline S722 degree 3 poles (32.2844, -386.4302) (32.4346, -386.2452) (32.7257, -385.8867) (33.1821, -385.8254) (33.4031, -385.7958) knots 0 0 0 0 0.068625 0.133023 0.133023 0.133023 0.133023
  spline S723 degree 3 poles (33.4031, -385.7958) (33.5681, -385.8042) (33.876, -385.8199) (34.1191, -386.0073) (34.2319, -386.0942) knots 0 0 0 0 0.048244 0.08997 0.08997 0.08997 0.08997
  spline S724 degree 3 poles (34.2319, -386.0942) (34.3161, -386.2166) (34.5056, -386.4915) (34.516, -386.8271) (34.5218, -387.0134) knots 0 0 0 0 0.043695 0.098195 0.098195 0.098195 0.098195
  line L541 (34.5218, -387.0134) -> (34.5218, -389.4997)
  line L542 (34.5218, -389.4997) -> (33.9113, -389.4998)
  line L543 (33.9113, -389.4998) -> (33.9113, -387.218)
  spline S725 degree 3 poles (33.9113, -387.218) (33.9112, -387.1118) (33.9112, -386.9325) (33.8688, -386.7586) (33.8516, -386.6877) knots 0 0 0 0 0.031711 0.053535 0.053535 0.053535 0.053535
  spline S726 degree 3 poles (33.8516, -386.6877) (33.8271, -386.636) (33.7773, -386.5306) (33.683, -386.4618) (33.635, -386.4268) knots 0 0 0 0 0.016863 0.034394 0.034394 0.034394 0.034394
  spline S727 degree 3 poles (33.635, -386.4268) (33.5793, -386.3979) (33.4638, -386.3382) (33.3339, -386.3314) (33.2666, -386.3279) knots 0 0 0 0 0.018597 0.038532 0.038532 0.038532 0.038532
  spline S728 degree 3 poles (33.2666, -386.3279) (33.1455, -386.3377) (32.9075, -386.3569) (32.7229, -386.5079) (32.6323, -386.582) knots 0 0 0 0 0.035532 0.069798 0.069798 0.069798 0.069798
  spline S729 degree 3 poles (32.6323, -386.582) (32.5589, -386.6887) (32.3918, -386.9318) (32.3842, -387.2288) (32.3799, -387.3954) knots 0 0 0 0 0.038079 0.086792 0.086792 0.086792 0.086792
  line L544 (32.3799, -387.3954) -> (32.3799, -389.4998)
  line L545 (32.3799, -389.4998) -> (31.766, -389.4998)
  line L546 (31.766, -389.4998) -> (31.766, -387.1464)
  spline S730 degree 3 poles (31.766, -387.1464) (31.7636, -387.0244) (31.7593, -386.8076) (31.6595, -386.6162) (31.6159, -386.5325) knots 0 0 0 0 0.036008 0.063954 0.063954 0.063954 0.063954
  spline S731 degree 3 poles (31.6159, -386.5325) (31.5537, -386.473) (31.4175, -386.3426) (31.2278, -386.3331) (31.1248, -386.3279) knots 0 0 0 0 0.025037 0.054812 0.054812 0.054812 0.054812
  spline S732 degree 3 poles (31.1248, -386.3279) (31.04, -386.3336) (30.8706, -386.3449) (30.7205, -386.4245) (30.6456, -386.4643) knots 0 0 0 0 0.025172 0.050327 0.050327 0.050327 0.050327
  spline S733 degree 3 poles (30.6456, -386.4643) (30.5769, -386.516) (30.4366, -386.6216) (30.3639, -386.7816) (30.3267, -386.8634) knots 0 0 0 0 0.025339 0.051812 0.051812 0.051812 0.051812
  spline S734 degree 3 poles (30.3267, -386.8634) (30.298, -386.9697) (30.2311, -387.2172) (30.229, -387.474) (30.2278, -387.6205) knots 0 0 0 0 0.032907 0.076633 0.076633 0.076633 0.076633
  line L547 (30.2278, -387.6205) -> (30.2278, -389.4998)
  line L548 (30.2278, -389.4998) -> (29.6139, -389.4998)
  line L549 (20.1494, -389.5) -> (20.1493, -388.3028)
  line L550 (20.1493, -388.3028) -> (17.9802, -388.3029)
  line L551 (17.9802, -388.3029) -> (17.9802, -387.7401)
  line L552 (17.9802, -387.7401) -> (20.2618, -384.5)
  line L553 (20.2618, -384.5) -> (20.7632, -384.5)
  line L554 (20.7632, -384.5) -> (20.7633, -387.7401)
  line L555 (20.7633, -387.7401) -> (21.4386, -387.7401)
  line L556 (21.4386, -387.7401) -> (21.4386, -388.3028)
  line L557 (21.4386, -388.3028) -> (20.7633, -388.3028)
  line L558 (20.7633, -388.3028) -> (20.7633, -389.5)
  line L559 (20.7633, -389.5) -> (20.1494, -389.5)
  line L560 (29.6186, -439.4991) -> (29.6184, -435.877)
  line L561 (29.6184, -435.877) -> (30.1675, -435.8769)
  line L562 (30.1675, -435.8769) -> (30.1675, -436.3851)
  spline S735 degree 3 poles (30.1675, -436.3851) (30.2294, -436.3005) (30.3543, -436.13) (30.5317, -436.015) (30.6211, -435.957) knots 0 0 0 0 0.031158 0.062835 0.062835 0.062835 0.062835
  spline S736 degree 3 poles (30.6211, -435.957) (30.7203, -435.9098) (30.9241, -435.8127) (31.1498, -435.801) (31.2657, -435.795) knots 0 0 0 0 0.032617 0.067048 0.067048 0.067048 0.067048
  spline S737 degree 3 poles (31.2657, -435.795) (31.3902, -435.7997) (31.6226, -435.8085) (31.8296, -435.9134) (31.9257, -435.962) knots 0 0 0 0 0.036859 0.068796 0.068796 0.068796 0.068796
  spline S738 degree 3 poles (31.9257, -435.962) (32.0053, -436.0238) (32.1663, -436.1484) (32.2478, -436.3351) (32.2889, -436.4293) knots 0 0 0 0 0.029725 0.060035 0.060035 0.060035 0.060035
  spline S739 degree 3 poles (32.2889, -436.4293) (32.4391, -436.2443) (32.7302, -435.8857) (33.1866, -435.8245) (33.4076, -435.7948) knots 0 0 0 0 0.068625 0.133023 0.133023 0.133023 0.133023
  spline S740 degree 3 poles (33.4076, -435.7948) (33.5727, -435.8032) (33.8805, -435.8189) (34.1236, -436.0063) (34.2364, -436.0932) knots 0 0 0 0 0.048244 0.08997 0.08997 0.08997 0.08997
  spline S741 degree 3 poles (34.2364, -436.0932) (34.3207, -436.2155) (34.5101, -436.4904) (34.5206, -436.826) (34.5264, -437.0123) knots 0 0 0 0 0.043695 0.098195 0.098195 0.098195 0.098195
  line L563 (34.5264, -437.0123) -> (34.5265, -439.4987)
  line L564 (34.5265, -439.4987) -> (33.916, -439.4987)
  line L565 (33.916, -439.4987) -> (33.9159, -437.217)
  spline S742 degree 3 poles (33.9159, -437.217) (33.9158, -437.1108) (33.9158, -436.9315) (33.8734, -436.7576) (33.8561, -436.6867) knots 0 0 0 0 0.031711 0.053535 0.053535 0.053535 0.053535
  spline S743 degree 3 poles (33.8561, -436.6867) (33.8317, -436.635) (33.7819, -436.5296) (33.6876, -436.4608) (33.6395, -436.4258) knots 0 0 0 0 0.016863 0.034394 0.034394 0.034394 0.034394
  spline S744 degree 3 poles (33.6395, -436.4258) (33.5838, -436.3969) (33.4684, -436.3372) (33.3384, -436.3304) (33.2712, -436.3269) knots 0 0 0 0 0.018597 0.038532 0.038532 0.038532 0.038532
  spline S745 degree 3 poles (33.2712, -436.3269) (33.15, -436.3367) (32.9121, -436.356) (32.7275, -436.5069) (32.6368, -436.581) knots 0 0 0 0 0.035532 0.069798 0.069798 0.069798 0.069798
  spline S746 degree 3 poles (32.6368, -436.581) (32.5635, -436.6877) (32.3964, -436.9309) (32.3888, -437.2278) (32.3845, -437.3945) knots 0 0 0 0 0.038079 0.086792 0.086792 0.086792 0.086792
  line L566 (32.3845, -437.3945) -> (32.3847, -439.4988)
  line L567 (32.3847, -439.4988) -> (31.7707, -439.4989)
  line L568 (31.7707, -439.4989) -> (31.7706, -437.1455)
  spline S747 degree 3 poles (31.7706, -437.1455) (31.7681, -437.0235) (31.7638, -436.8067) (31.6641, -436.6153) (31.6205, -436.5316) knots 0 0 0 0 0.036008 0.063954 0.063954 0.063954 0.063954
  spline S748 degree 3 poles (31.6205, -436.5316) (31.5582, -436.4721) (31.422, -436.3417) (31.2323, -436.3322) (31.1293, -436.327) knots 0 0 0 0 0.025037 0.054812 0.054812 0.054812 0.054812
  spline S749 degree 3 poles (31.1293, -436.327) (31.0445, -436.3327) (30.8751, -436.3441) (30.7251, -436.4237) (30.6501, -436.4635) knots 0 0 0 0 0.025172 0.050327 0.050327 0.050327 0.050327
  spline S750 degree 3 poles (30.6501, -436.4635) (30.5815, -436.5152) (30.4412, -436.6208) (30.3684, -436.7808) (30.3313, -436.8626) knots 0 0 0 0 0.025339 0.051812 0.051812 0.051812 0.051812
  spline S751 degree 3 poles (30.3313, -436.8626) (30.3026, -436.9689) (30.2357, -437.2164) (30.2336, -437.4732) (30.2324, -437.6197) knots 0 0 0 0 0.032907 0.076633 0.076633 0.076633 0.076633
  line L569 (30.2324, -437.6197) -> (30.2325, -439.499)
  line L570 (30.2325, -439.499) -> (29.6186, -439.4991)
  line L571 (20.1541, -439.4998) -> (20.154, -438.3027)
  line L572 (20.154, -438.3027) -> (17.9848, -438.3028)
  line L573 (17.9848, -438.3028) -> (17.9848, -437.7401)
  line L574 (17.9848, -437.7401) -> (20.2663, -434.4998)
  line L575 (20.2663, -434.4998) -> (20.7676, -434.4997)
  line L576 (20.7676, -434.4997) -> (20.7679, -437.7398)
  line L577 (20.7679, -437.7398) -> (21.4432, -437.7398)
  line L578 (21.4432, -437.7398) -> (21.4432, -438.3026)
  line L579 (21.4432, -438.3026) -> (20.7679, -438.3026)
  line L580 (20.7679, -438.3026) -> (20.768, -439.4997)
  line L581 (20.768, -439.4997) -> (20.1541, -439.4998)
  line L582 (29.5119, -489.4998) -> (29.5118, -485.8777)
  line L583 (29.5118, -485.8777) -> (30.0609, -485.8777)
  line L584 (30.0609, -485.8777) -> (30.0609, -486.3859)
  spline S752 degree 3 poles (30.0609, -486.3859) (30.1228, -486.3013) (30.2477, -486.1308) (30.4251, -486.0158) (30.5145, -485.9579) knots 0 0 0 0 0.031158 0.062835 0.062835 0.062835 0.062835
  spline S753 degree 3 poles (30.5145, -485.9579) (30.6137, -485.9106) (30.8176, -485.8135) (31.0433, -485.8018) (31.1591, -485.7958) knots 0 0 0 0 0.032617 0.067048 0.067048 0.067048 0.067048
  spline S754 degree 3 poles (31.1591, -485.7958) (31.2836, -485.8006) (31.516, -485.8094) (31.723, -485.9143) (31.8191, -485.9629) knots 0 0 0 0 0.036859 0.068796 0.068796 0.068796 0.068796
  spline S755 degree 3 poles (31.8191, -485.9629) (31.8988, -486.0247) (32.0597, -486.1493) (32.1412, -486.336) (32.1824, -486.4302) knots 0 0 0 0 0.029725 0.060035 0.060035 0.060035 0.060035
  spline S756 degree 3 poles (32.1824, -486.4302) (32.3325, -486.2452) (32.6236, -485.8867) (33.0801, -485.8254) (33.301, -485.7958) knots 0 0 0 0 0.068625 0.133023 0.133023 0.133023 0.133023
  spline S757 degree 3 poles (33.301, -485.7958) (33.4661, -485.8042) (33.774, -485.8199) (34.0171, -486.0073) (34.1298, -486.0942) knots 0 0 0 0 0.048244 0.08997 0.08997 0.08997 0.08997
  spline S758 degree 3 poles (34.1298, -486.0942) (34.2141, -486.2165) (34.4035, -486.4914) (34.414, -486.8271) (34.4197, -487.0134) knots 0 0 0 0 0.043695 0.098195 0.098195 0.098195 0.098195
  line L585 (34.4197, -487.0134) -> (34.4198, -489.4997)
  line L586 (34.4198, -489.4997) -> (33.8093, -489.4998)
  line L587 (33.8093, -489.4998) -> (33.8092, -487.218)
  spline S759 degree 3 poles (33.8092, -487.218) (33.8092, -487.1118) (33.8092, -486.9325) (33.7668, -486.7586) (33.7495, -486.6877) knots 0 0 0 0 0.031711 0.053535 0.053535 0.053535 0.053535
  spline S760 degree 3 poles (33.7495, -486.6877) (33.7251, -486.636) (33.6753, -486.5306) (33.581, -486.4618) (33.533, -486.4268) knots 0 0 0 0 0.016863 0.034394 0.034394 0.034394 0.034394
  spline S761 degree 3 poles (33.533, -486.4268) (33.4772, -486.3979) (33.3618, -486.3382) (33.2318, -486.3314) (33.1646, -486.3279) knots 0 0 0 0 0.018597 0.038532 0.038532 0.038532 0.038532